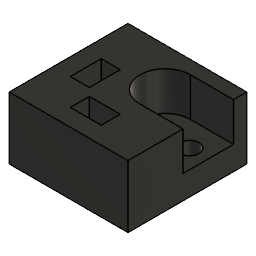
Front Base Upper (Autodesk Fusion 360 design; units mm, degrees)
Autodesk Fusion 360 part; units mm, degrees
sketch "スケッチ1" plane through (0, 0, 0) normal (0, 0, 1) x (1, 0, 0)
  line L0 (0, 0) -> (20, 0)
  line L1 (20, 0) -> (20, 20)
  line L2 (20, 20) -> (0, 20)
  line L3 (0, 20) -> (0, 0)
  dimension "d1" = 20
  dimension "d2" = 20
  constraint horizontal L0
  constraint vertical L1
  constraint horizontal L2
  constraint vertical L3
  constraint coincident L0.start L3.end
  measures "d1" distance of L1.end L2.end
  measures "d2" distance of L0.start L2.end
extrude "押し出し1" add sketch "スケッチ1" along normal blind 21
sketch "スケッチ2" plane through (20, 0, 0) normal (1, 0, 0) x (0, 1, 0)
  line L0 (0, 0) -> (20, 0)
  line L1 (20, 0) -> (20, 21)
  line L2 (20, 21) -> (0, 21)
  line L3 (0, 21) -> (0, 0)
  circle A0 centre (5, 5) radius 1.15
  dimension "d5" = 2.3
  dimension "d8" = 5
  dimension "d11" = 5
  measures "d5" diameter of A0
  measures "d8" distance of L3 A0.centre
  measures "d11" distance of L0 A0.centre
extrude "押し出し2" cut sketch "スケッチ2" against normal blind 25 contours A0
sketch "スケッチ7" plane through (0, 0, 21) normal (0, 0, 1) x (-1, 0, 0)
  line L0 (0, -20) -> (0, 0)
  line L1 (0, 0) -> (-20, 0)
  line L2 (-20, 0) -> (-20, -20)
  line L3 (-20, -20) -> (0, -20)
  line L4 (-12.75, -17.75) -> (-20, -17.75)
  line L5 (-20, -17.75) -> (-20, -9.25)
  line L6 (-20, -9.25) -> (-12.75, -9.25)
  line L7 (-8.5, -13.5) -> (-20, -13.5)
  circle A0 centre (-12.85, -13.5) radius 1.6
  circle A1 centre (-16.85, -13.5) radius 1.6
  arc A2 (-12.75, -17.75) -> (-8.5, -13.5) centre (-12.75, -13.5) ccw
  arc A3 (-8.5, -13.5) -> (-12.75, -9.25) centre (-12.75, -13.5) ccw
  point P0 (-8.5, -17.75)
  point P1 (-8.5, -9.25)
  dimension "d16" = 8.5
  dimension "d17" = 11.5
  dimension "d18" = 3.2
  dimension "d19" = 3.2
  dimension "d20" = 4
  dimension "d21" = 4.35
  dimension "d22" = 4.25
  dimension "d23" = 4.25
  dimension "d24" = 4.25
  constraint horizontal L4
  constraint vertical L5
  constraint horizontal L6
  constraint coincident L2 L5.end
  constraint coincident L5 L7.end
  constraint perpendicular L5 L7
  constraint coincident L7 A0.centre
  constraint coincident L7 A1.centre
  constraint coincident P0 L4
  constraint tangent L4 A2
  constraint coincident P1 L6
  constraint tangent L6 A3
  constraint coincident L7.start A2.end
  measures "d16" distance of P0 P1
  measures "d17" distance of P0 L4.end
  measures "d18" diameter of A0
  measures "d19" diameter of A1
  measures "d20" distance of A0.centre A1.centre
  measures "d21" distance of L7.start A0.centre
  measures "d22" radius of A2
  measures "d23" distance of L4 L7
  measures "d24" radius of A3
extrude "押し出し4" cut sketch "スケッチ7" against normal blind 6.5 contours L2 L4 L5 L7 A0 A1 A2 | L2 L5 L6 L7 A0 A1 A3
extrude "押し出し5" cut 2 faces at (12.2215, 13.3267, 21) (16.1057, 13.3074, 21) along direction (0, 0, -1) blind 26
sketch "スケッチ11" plane through (20, 0, 0) normal (1, 0, 0) x (0, 1, 0)
  line L0 (17.75, 21) -> (17.75, 14.5)
  line L1 (17.75, 14.5) -> (9.25, 14.5)
  line L2 (9.25, 14.5) -> (9.25, 21)
  line L3 (9.25, 21) -> (0, 21)
  line L4 (0, 21) -> (0, 0)
  line L5 (0, 0) -> (20, 0)
  line L6 (20, 0) -> (20, 21)
  line L7 (20, 21) -> (17.75, 21)
  circle A0 centre (5, 5) radius 1.15
  line L8 (0, 10.5) -> (20, 10.5)
  line L9 (20, 10.5) -> (20, 0)
  line L10 (20, 0) -> (0, 0)
  line L11 (0, 0) -> (0, 10.5)
  dimension "d34" = 4
  constraint horizontal L8
  constraint vertical L9
  constraint horizontal L10
  constraint vertical L11
  constraint coincident L5.end L6.start
  constraint coincident L4 L8.start
  measures "d34" distance of L1 L8
extrude "押し出し8" cut sketch "スケッチ11" against normal blind 32 contours L4 L5 L6 L8 L9 L10 L11
sketch "スケッチ12" plane through (0, 0, 21) normal (0, 0, 1) x (-1, 0, 0)
  line L0 (-12.75, -17.75) -> (-20, -17.75)
  line L1 (-20, -17.75) -> (-20, -20)
  line L2 (-20, -20) -> (0, -20)
  line L3 (0, -20) -> (0, 0)
  line L4 (0, 0) -> (-20, 0)
  line L5 (-20, 0) -> (-20, -9.25)
  line L6 (-20, -9.25) -> (-12.75, -9.25)
  arc A0 (-12.75, -17.75) -> (-12.75, -9.25) centre (-12.75, -13.5) ccw
  line L7 (-2.9, -12.6) -> (-6.1, -12.6)
  line L8 (-6.1, -12.6) -> (-6.1, -7.4)
  line L9 (-6.1, -7.4) -> (-2.9, -7.4)
  line L10 (-2.9, -7.4) -> (-2.9, -12.6)
  line L11 (-12.6, -2.9) -> (-7.4, -2.9)
  line L12 (-7.4, -2.9) -> (-7.4, -6.1)
  line L13 (-7.4, -6.1) -> (-12.6, -6.1)
  line L14 (-12.6, -6.1) -> (-12.6, -2.9)
  dimension "d37" = 2.9
  dimension "d38" = 5.2
  dimension "d39" = 3.2
  dimension "d40" = 7.4
  dimension "d41" = 3.2
  dimension "d42" = 5.2
  dimension "d43" = 2.9
  dimension "d44" = 7.4
  constraint horizontal L7
  constraint vertical L8
  constraint horizontal L9
  constraint vertical L10
  constraint horizontal L11
  constraint vertical L12
  constraint horizontal L13
  constraint vertical L14
  measures "d37" distance of L4 L11
  measures "d38" distance of L12.end L13.end
  measures "d39" distance of L11.start L13.end
  measures "d40" distance of L5 L14
  measures "d41" distance of L7.start L7.end
  measures "d42" distance of L7.end L8.end
  measures "d43" distance of L3 L10
  measures "d44" distance of L2 L7
extrude "押し出し9" cut sketch "スケッチ12" against normal blind 22 contours L7 L8 L9 L10 | L11 L12 L13 L14
equation "d40 = 10 mm - 2.6 mm"
